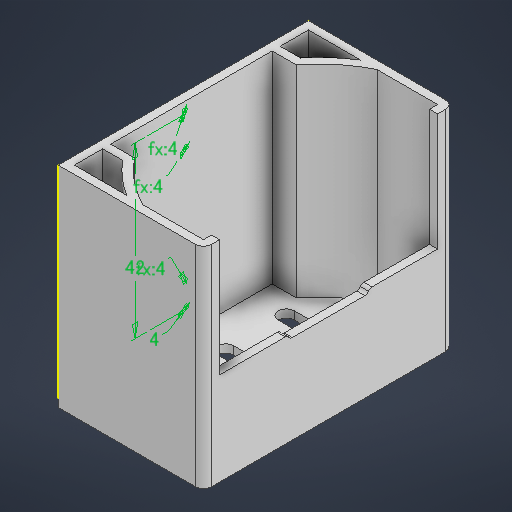
# Autodesk Inventor part: default
Saved by Autodesk Inventor 2025.2 (Build 292293000, 293)
## iProperties
Created: 2024-07-26
Part Number: default
Material: 一般
Document SubType Name: Modeling
Designer: ktamu
Density: 1 g/cm^3
Appearance: 既定
Author: ktamu
Autodesk Inventor part; units mm, degrees
ref_plane "YZ Plane" through (0, 0, 0) normal (1, 0, 0) x (0, 1, 0)
ref_plane "XZ Plane" through (0, 0, 0) normal (0, 1, 0) x (-1, 0, 0)
ref_plane "XY Plane" through (0, 0, 0) normal (0, 0, 1) x (1, 0, 0)
sketch "スケッチ1" plane through (0, 0, 0) normal (0, 1, 0) x (-1, 0, 0)
  line L0 (16, 29) -> (-16, 29)
  line L1 (-16, 29) -> (-16, -29)
  line L2 (-16, -29) -> (16, -29)
  line L3 (16, -29) -> (16, 29)
  line L4 (16, 29) -> (-16, -29) construction
  line L5 (-16, 29) -> (16, -29) construction
  line L6 (18, 31) -> (-18, 31)
  line L7 (-18, 31) -> (-18, -31)
  line L8 (-18, -31) -> (18, -31)
  line L9 (18, -31) -> (18, 31)
  arc A0 (-1, -29) -> (-1, 29) centre (-15.3611, 0) ccw
  line L10 (0, 0) -> (6.445, 0)
  arc A1 (-0.1124, -30.7923) -> (-0.1124, 30.7923) centre (-15.3611, 0) ccw
  line L11 (16, 20) -> (10.0798, 20)
  line L12 (10.0798, 20) -> (10.0798, -20)
  line L13 (10.0798, -20) -> (16, -20)
  line L14 (16, -20) -> (16, 20)
  line L15 (-16, 10) -> (-18, 10)
  line L16 (-18, 10) -> (-18, -10)
  line L17 (-18, -10) -> (-16, -10)
  line L18 (-16, -10) -> (-16, 10)
  line L19 (-12.375, 31) -> (-12.375, 29)
  line L20 (-11.6594, -29) -> (-11.6594, -31)
  line L21 (10.9703, 20) -> (10.9703, 22)
  line L22 (10.9703, 22) -> (16, 22)
  line L23 (16, -20) -> (10.0798, -20)
  line L24 (10.9703, -20) -> (10.9703, -22)
  line L25 (10.9703, -22) -> (16, -22)
  line L26 (-16, 27) -> (-18, 27)
  line L27 (-16, -27) -> (-18, -27)
  point P0 (16, -20)
  point P1 (-17, 10)
  point P2 (12.5796, 20)
  point P3 (3.0695, 29)
  point P4 (3.0695, -29)
  point P5 (12.5796, -20)
  point P6 (11.0337, -22)
  point P7 (11.0337, 22)
  dimension "d0" = 32
  dimension "d1" = 58
  dimension "d2" = 2
  dimension "d3" = 15
  dimension "d4" = 15
  dimension "d5" = 20
  dimension "d6" = 20
  dimension "d7" = 2
  dimension "d8" = 20
  dimension "d16" = 2
  dimension "d17" = 4
  constraints: 56 end point, 15 point on line, 9 perpendicular, 8 parallel, 5 point on circle, 5 symmetric about line, 4 horizontal, 3 midpoint, 2 centre point, 4 other
  measures "d0" distance of L2.end L1.end
  measures "d1" distance of L1.end L0.end
  measures "d2" distance between parallel lines of L3 L9
  measures "d3" distance from line of L1 A0.start
  measures "d4" distance from line of L1 A0.end
  measures "d5" distance from line of L10 L11.start
  measures "d6" distance from line of L10 point (16, -20)
  measures "d7" radial gap between concentric circles of A0 A1
  measures "d8" distance from line of L17 point (-17, 10)
  measures "d16" distance of L21.start L21.end
  measures "d17" distance between parallel lines of L6 L26
extrude "押し出し1" add sketch "スケッチ1" along normal blind 20 contours L1 L17 L7 L15
extrude "押し出し2" add sketch "スケッチ1" along normal blind 21 contours L0 L1 L26 L7 L6 L19 | L1 L15 L7 L26 | L20 L8 L7 L27 L1 L2 | L1 L27 L7 L17
fillet "フィレット1" radius 1 4 edges at (17, 21, -10) (17, 20, -10) (17, 21, 10) (17, 20, 10)
extrude "押し出し3" add sketch "スケッチ1" along normal blind 50 contours L0 L19 L6 L9 A1 L3 | L0 A1 L22 L21 L11 A0 | A1 L11 L21 L22 | A0 L3 | L3 A1 L9 A0 | L13 L24 L25 A1 L2 A0 | L2 L3 A1 L9 L8 L20 | L13 A1 L25 L24
extrude "押し出し4" add sketch "スケッチ1" along normal blind 50 contours L0 L1 L26 L7 L6 L19 | L20 L8 L7 L27 L1 L2
extrude "押し出し5" add sketch "スケッチ1" along normal blind 50 contours L22 L3 L11 A1 | L13 L3 L25 A1
fillet "フィレット2" radius 2 2 edges at (18, 25, 31) (18, 25, -31)
sketch "スケッチ2" plane through (-18, 0, -31) normal (-1, 0, 0) x (0, 0, 1)
  line L0 (31, 45.2367) -> (31, 3.2367)
  line L1 (0, 0) -> (0, 50) projected
  line L2 (0, 0) -> (0, 13.3376)
  line L3 (62, 50) -> (62, 0) projected
  line L4 (62, 0) -> (62, 13.3376)
  circle A0 centre (31, 3.2367) radius 2
  circle A1 centre (31, 45.2367) radius 2
  circle A2 centre (31, 37.4238) radius 2
  circle A3 centre (31, 10.2787) radius 2
  line L5 (29, 45.2367) -> (29, 37.4238)
  line L6 (33, 37.4238) -> (33, 45.2367)
  line L7 (29, 10.2787) -> (29, 3.2367)
  line L8 (33, 3.2367) -> (33, 10.2787)
  point P0 (31, 0)
  dimension "d23" = 42
  dimension "d24" = 4
  dimension "d25" = 4
  dimension "d26" = 4
  dimension "d27" = 4
  constraints: 14 end point, 8 point on circle, 8 point on line, 4 centre point, 2 coincident, 2 tangent, 2 vertical, 1 symmetric about line
  measures "d23" distance of L0.start L0.end
  measures "d24" diameter of A0
  measures "d25" diameter of A1
  measures "d26" diameter of A2
  measures "d27" diameter of A3
sketch "スケッチ3" plane through (0, 0, 0) normal (0, -1, 0) x (1, 0, 0)
  line L0 (7.5, 2) -> (-7.5, 2)
  line L1 (-7.5, 2) -> (-7.5, -2)
  line L2 (-7.5, -2) -> (7.5, -2)
  line L3 (7.5, -2) -> (7.5, 2)
  line L4 (7.5, 2) -> (-7.5, -2) construction
  line L5 (-7.5, 2) -> (7.5, -2) construction
  arc A0 (7.5, -2) -> (7.5, 2) centre (7.5, 0) ccw
  arc A1 (-7.5, 2) -> (-7.5, -2) centre (-7.5, 0) ccw
  line L6 (7.5, 17) -> (-7.5, 17)
  line L7 (-7.5, 17) -> (-7.5, 13)
  line L8 (-7.5, 13) -> (7.5, 13)
  line L9 (7.5, 13) -> (7.5, 17)
  line L10 (7.5, 17) -> (-7.5, 13) construction
  line L11 (-7.5, 17) -> (7.5, 13) construction
  arc A2 (7.5, 13) -> (7.5, 17) centre (7.5, 15) ccw
  arc A3 (-7.5, 17) -> (-7.5, 13) centre (-7.5, 15) ccw
  line L12 (7.5, -13) -> (-7.5, -13)
  line L13 (-7.5, -13) -> (-7.5, -17)
  line L14 (-7.5, -17) -> (7.5, -17)
  line L15 (7.5, -17) -> (7.5, -13)
  line L16 (7.5, -13) -> (-7.5, -17) construction
  line L17 (-7.5, -13) -> (7.5, -17) construction
  arc A4 (7.5, -17) -> (7.5, -13) centre (7.5, -15) ccw
  arc A5 (-7.5, -13) -> (-7.5, -17) centre (-7.5, -15) ccw
  line L18 (-18, 31) -> (16, 31) projected
  arc A6 (18, 29) -> (16, 31) centre (16, 29) ccw projected
  line L19 (18, 29) -> (18, -29) projected
  arc A7 (16, -31) -> (18, -29) centre (16, -29) ccw projected
  line L20 (16, -31) -> (-18, -31) projected
  line L21 (-18, -31) -> (-18, 31) projected
  line L22 (-3.0695, 29) -> (-16, 29) projected
  arc A8 (-3.0695, 29) -> (-11.0337, 22) centre (15.3611, 0) ccw projected
  line L23 (-16, 22) -> (-11.0337, 22) projected
  line L24 (-16, 29) -> (-16, 22) projected
  line L25 (-11.0337, -22) -> (-16, -22) projected
  arc A9 (-11.0337, -22) -> (-3.0695, -29) centre (15.3611, 0) ccw projected
  line L26 (-16, -29) -> (-3.0695, -29) projected
  line L27 (-16, -22) -> (-16, -29) projected
  point P0 (0, 0)
  point P1 (0, 15)
  point P2 (0, -15)
  dimension "d28" = 15
  dimension "d29" = 4
  dimension "d32" = 15
  constraints: 36 end point, 12 point on circle, 6 centre point, 4 midpoint, 2 parallel, 1 collinear, 1 horizontal, 1 perpendicular, 1 vertical, 29 other
  measures "d28" distance of L2.end L1.end
  measures "d29" distance of L1.end L0.end
  measures "d32" distance of L0.start L6.start
extrude "押し出し6" add sketch "スケッチ3" along normal blind 2
equation "\"d4\" = d3"
equation "\"d6\" = d5"
equation "\"d25\" = d24"
equation "\"d26\" = d25"
equation "\"d27\" = d26"
